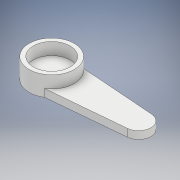
# Autodesk Inventor part: learnbotBrazoServo
Saved by Autodesk Inventor 2017 (Build 210142000, 142)
## iProperties
Part Number: learnbotBrazoServo
Material: Genérico
Document SubType Name: Modeling
Designer: rober
Density: 1 g/cm^3
Appearance: Valor por defecto
Author: rober
Autodesk Inventor part; units mm, degrees
ref_plane "YZ Plane" through (0, 0, 0) normal (1, 0, 0) x (0, 1, 0)
ref_plane "XZ Plane" through (0, 0, 0) normal (0, 1, 0) x (-1, 0, 0)
ref_plane "XY Plane" through (0, 0, 0) normal (0, 0, 1) x (1, 0, 0)
sketch "Boceto1" plane through (0, 0, 0) normal (0, 0, 1) x (1, 0, 0)
  arc A0 (0.2295, 0.2896) -> (0.1967, -0.3128) centre (0, 0) ccw
  arc A1 (1.4408, -0.1992) -> (1.4375, 0.1994) centre (1.4226, 0) ccw
  line L0 (0.2295, 0.2896) -> (1.4375, 0.1994)
  line L1 (0.1967, -0.3128) -> (1.4408, -0.1992)
  circle A2 centre (0, 0) radius 0.3
  constraints: 4 end point, 4 point on circle, 3 centre point
extrude "Extrusión1" add sketch "Boceto1" along normal blind 0.125 contours L0 A1 L1 A0 | A2
sketch "Boceto2" plane through (0, 0, 0.125) normal (0, 0, 1) x (1, 0, 0)
  arc A0 (0.2295, 0.2896) -> (0.1967, -0.3128) centre (0, 0) ccw
  arc A1 (1.4408, -0.1992) -> (1.4375, 0.1994) centre (1.4226, 0) ccw
  line L0 (0.2295, 0.2896) -> (1.4375, 0.1994)
  line L1 (0.1967, -0.3128) -> (1.4408, -0.1992)
  circle A2 centre (0, 0) radius 0.3
  circle A3 centre (0, 0) radius 0.3695
  constraints: 4 end point, 4 point on circle, 3 centre point, 1 coincident, 3 other
extrude "Extrusión2" add sketch "Boceto2" along normal blind 0.2 contours A3 A0
